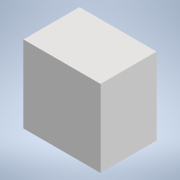
# Autodesk Inventor part: base
Saved by Autodesk Inventor 2020 (Build 240168000, 168)
## iProperties
Created: 2020-03-06
Part Number: base
Material: Generic
Document SubType Name: Modeling
Designer: udvarhelyi
Density: 1 g/cm^3
Appearance: Default
Author: udvarhelyi
Autodesk Inventor part; units mm, degrees
ref_plane "YZ Plane" through (0, 0, 0) normal (1, 0, 0) x (0, 1, 0)
ref_plane "XZ Plane" through (0, 0, 0) normal (0, 1, 0) x (-1, 0, 0)
ref_plane "XY Plane" through (0, 0, 0) normal (0, 0, 1) x (1, 0, 0)
sketch "Sketch1" plane through (0, 0, 0) normal (0, 1, 0) x (-1, 0, 0)
  line L0 (23.4545, 19) -> (23.4545, 22)
  line L1 (18.9091, 22) -> (18.9091, 19)
  line L2 (14.3636, 19) -> (14.3636, 22)
  line L3 (9.8182, 22) -> (9.8182, 19)
  line L4 (5.2727, 19) -> (5.2727, 22)
  line L5 (0.7273, 22) -> (0.7273, 19)
  line L6 (-3.8182, 19) -> (-3.8182, 22)
  line L7 (-8.3636, 22) -> (-8.3636, 19)
  line L8 (-12.9091, 19) -> (-12.9091, 22)
  line L9 (-17.4545, 22) -> (-17.4545, 19)
  line L10 (-22, 15) -> (-19, 15)
  line L11 (-19, 3) -> (-22, 3)
  line L12 (-19, -9) -> (-22, -9)
  line L13 (-22, -21) -> (-19, -21)
  line L14 (-17.4545, -25) -> (-17.4545, -28)
  line L15 (-12.9091, -28) -> (-12.9091, -25)
  line L16 (-8.3636, -25) -> (-8.3636, -28)
  line L17 (-3.8182, -28) -> (-3.8182, -25)
  line L18 (0.7273, -28) -> (0.7273, -25)
  line L19 (5.2727, -25) -> (5.2727, -28)
  line L20 (23.4545, -28) -> (23.4545, -25)
  line L21 (18.9091, -25) -> (18.9091, -28)
  line L22 (14.3636, -28) -> (14.3636, -25)
  line L23 (9.8182, -25) -> (9.8182, -28)
  line L24 (28, -21) -> (25, -21)
  line L25 (25, 15) -> (28, 15)
  line L26 (28, 3) -> (25, 3)
  line L27 (18.9091, -28) -> (23.4545, -28)
  line L28 (9.8182, -28) -> (14.3636, -28)
  line L29 (0.7273, -28) -> (5.2727, -28)
  line L30 (28, -21) -> (28, -17)
  line L31 (28, 3) -> (28, 7)
  line L32 (28, 11) -> (28, 15)
  line L33 (23.4545, 22) -> (18.9091, 22)
  line L34 (14.3636, 22) -> (9.8182, 22)
  line L35 (5.2727, 22) -> (0.7273, 22)
  line L36 (-3.8182, 22) -> (-8.3636, 22)
  line L37 (-12.9091, 22) -> (-17.4545, 22)
  line L38 (-19, 15) -> (-19, 11)
  line L39 (-19, 7) -> (-19, 3)
  line L40 (-22, 3) -> (-22, -1)
  line L41 (-22, 19) -> (-22, 15)
  line L42 (-17.4545, -28) -> (-12.9091, -28)
  line L43 (-8.3636, -28) -> (-3.8182, -28)
  line L44 (-19, -9) -> (-19, -13)
  line L45 (-19, -17) -> (-19, -21)
  line L46 (-22, -5) -> (-22, -9)
  line L47 (-22, -21) -> (-22, -25)
  line L48 (-22, -25) -> (-17.4545, -25)
  line L49 (-12.9091, -25) -> (-8.3636, -25)
  line L50 (-3.8182, -25) -> (0.7273, -25)
  line L51 (5.2727, -25) -> (9.8182, -25)
  line L52 (14.3636, -25) -> (18.9091, -25)
  line L53 (23.4545, -25) -> (25, -25)
  line L54 (25, -25) -> (25, -21)
  line L55 (25, -1) -> (25, 3)
  line L56 (25, 15) -> (25, 19)
  line L57 (25, 19) -> (23.4545, 19)
  line L58 (18.9091, 19) -> (14.3636, 19)
  line L59 (9.8182, 19) -> (5.2727, 19)
  line L60 (0.7273, 19) -> (-3.8182, 19)
  line L61 (-8.3636, 19) -> (-12.9091, 19)
  line L62 (-17.4545, 19) -> (-22, 19)
  line L63 (28, -13) -> (28, -9)
  line L64 (28, -9) -> (25, -9)
  line L65 (25, -9) -> (25, -5)
  line L66 (-19, -17) -> (-19, -13)
  line L67 (-22, -5) -> (-22, -1)
  line L68 (-19, 7) -> (-19, 11)
  line L69 (28, -17) -> (28, -13)
  line L70 (25, -5) -> (25, -1)
  line L71 (28, 7) -> (28, 11)
  point P0 (0, 0)
  point P1 (-219, 16.6364)
  point P2 (-222, -22.6364)
  point P3 (228, -22.6364)
  point P4 (-11.5, 9)
  point P5 (-11.5, 6.8182)
  point P6 (-14.5, 0.2727)
  point P7 (-11.5, -6.2727)
  point P8 (20.5, -12.8182)
  point P9 (20.5, -10.6364)
  point P10 (17.5, -3.0455)
  point P11 (17.5, -2.9545)
  point P12 (-11.5, 6.8182)
  point P13 (-14.5, 6.8182)
  point P14 (-14.5, 5)
  point P15 (-14.5, 9)
  dimension "d1" = 47
  dimension "d3" = 44
  dimension "d5" = 25
  dimension "d6" = 25
  dimension "d9" = 3
  dimension "d15" = 3
  dimension "d16" = 3
  dimension "d17" = 3
  dimension "d18" = 12
  dimension "d19" = 12
  dimension "d20" = 12
  dimension "d21" = 4
  dimension "d23" = 4.5454
  constraints: 167 perpendicular, 144 end point, 89 parallel, 44 collinear, 13 equal length, 6 horizontal, 3 vertical
  measures "d1" distance of L47.end L53.end
  measures "d3" distance of L53.end L56.end
  measures "d5" horizontal distance of L53.end point (0, 0)
  measures "d6" horizontal distance of L53.end point (0, 0)
  measures "d9" distance of L13.start L13.end
  measures "d15" distance of L20.start L20.end
  measures "d16" distance of L0.start L0.end
  measures "d17" distance of L24.start L24.end
  measures "d18" distance between parallel lines of L64 L24
  measures "d19" distance between parallel lines of L26 L64
  measures "d20" distance between parallel lines of L25 L26
  measures "d21" distance of L53.end L24.end
  measures "d23" distance of L23.end L22.start
extrude "Extrusion1" add sketch "Sketch1" along normal blind 3
equation "\"d1\" = wt - tt"
equation "\"d3\" = -2 * tt + ht"
equation "\"d5\" = 0.5 * ht"
equation "\"d6\" = 0.5 * wt"
equation "\"d9\" = tt"
equation "\"d15\" = tt"
equation "\"d16\" = tt"
equation "\"d17\" = tt"
equation "\"d18\" = 0.272727 * ht - 0.545455 * tt"
equation "\"d19\" = d18"
equation "\"d20\" = d18"
equation "\"d21\" = -0.181818 * tt + 0.0909091 * ht"
equation "\"d23\" = 0.0909091 * wt"
equation "\"d13\" = tt"
equation "\"wt\" = 50"
equation "\"tt\" = 3"
equation "\"tol\" = 0"
equation "\"tiroir\" = 25.4"
equation "\"nHoles\" = 101.6"
equation "\"shelfH\" = 35"
equation "\"d0\" = 0.5 * wt"
equation "\"d2\" = 0.5 * lt"
equation "\"d4\" = tt"
equation "\"ht\" = 50"
equation "\"lt\" = 50"
body "Solid1"
